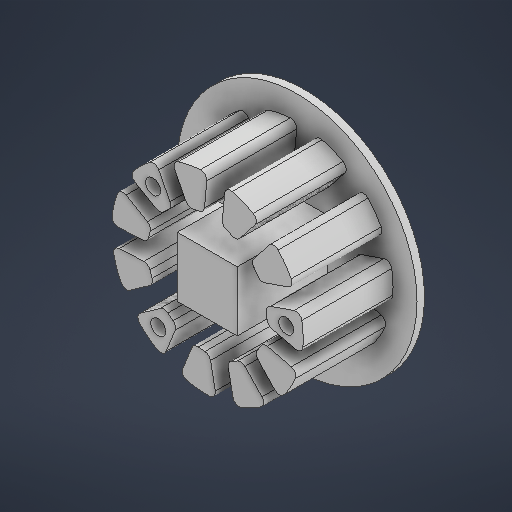
# Autodesk Inventor part: новая сиська 5-26
Saved by Autodesk Inventor 2025 (Build 290162000, 162)
## iProperties
Created: 2025-10-01
Part Number: новая сиська 5-26
Material: Типовые
Document SubType Name: Modeling
Designer: GameHD
Density: 1 g/cm^3
Appearance: По умолчанию
Author: GameHD
Autodesk Inventor part; units mm, degrees
ref_plane "YZ Plane" through (0, 0, 0) normal (1, 0, 0) x (0, 1, 0)
ref_plane "XZ Plane" through (0, 0, 0) normal (0, 1, 0) x (-1, 0, 0)
ref_plane "XY Plane" through (0, 0, 0) normal (0, 0, 1) x (1, 0, 0)
sketch "Эскиз1" plane through (0, 0, 0) normal (0, 0, 1) x (1, 0, 0)
  arc A0 (18.0451, 11.2945) -> (16.7558, 13.0882) centre (1.2512, 0.5834) ccw
  arc A1 (16.735, 15.5731) -> (16.7558, 13.0882) centre (18.3126, 14.3437) ccw
  line L0 (16.735, 15.5731) -> (21.7996, 22.0722)
  arc A2 (24.8522, 22.1935) -> (21.7996, 22.0722) centre (23.3772, 20.8429) ccw
  arc A3 (29.2559, 16.067) -> (24.8522, 22.1935) centre (1.2512, 0.5834) ccw
  arc A4 (28.1681, 13.2122) -> (29.2559, 16.067) centre (27.5056, 15.0993) ccw
  line L1 (28.1681, 13.2122) -> (20.3938, 10.4829)
  arc A5 (18.0451, 11.2945) -> (20.3938, 10.4829) centre (19.7313, 12.37) ccw
  line L2 (-17.9086, -9.4147) -> (-24.6202, -14.1941)
  arc A6 (-27.58, -13.4373) -> (-24.6202, -14.1941) centre (-25.7803, -12.5649) ccw
  arc A7 (-30.0477, -6.3074) -> (-27.58, -13.4373) centre (1.2153, 0.5208) ccw
  arc A8 (-28.189, -3.8829) -> (-30.0477, -6.3074) centre (-28.0938, -5.8806) ccw
  line L3 (-28.189, -3.8829) -> (-19.9588, -3.4908)
  arc A9 (-17.9403, -4.9402) -> (-19.9588, -3.4908) centre (-19.8637, -5.4886) ccw
  arc A10 (-17.9403, -4.9402) -> (-17.2178, -7.0277) centre (1.2153, 0.5208) ccw
  arc A11 (-17.9086, -9.4147) -> (-17.2178, -7.0277) centre (-19.0687, -7.7856) ccw
  line L4 (-9.5011, -18.1766) -> (-12.5634, -25.8259)
  arc A12 (-15.4625, -26.7894) -> (-12.5634, -25.8259) centre (-14.4202, -25.0825) ccw
  arc A13 (-21.3932, -22.1255) -> (-15.4625, -26.7894) centre (1.2153, 0.5208) ccw
  arc A14 (-21.1403, -19.0809) -> (-21.3932, -22.1255) centre (-19.9802, -20.7101) ccw
  line L5 (-21.1403, -19.0809) -> (-14.4286, -14.3016)
  arc A15 (-11.9469, -14.4296) -> (-14.4286, -14.3016) centre (-13.2685, -15.9307) ccw
  arc A16 (-11.9469, -14.4296) -> (-10.2106, -15.7951) centre (1.2153, 0.5208) ccw
  arc A17 (-9.5011, -18.1766) -> (-10.2106, -15.7951) centre (-11.3579, -17.4333) ccw
  line L6 (-15.7668, 13.7891) -> (-22.9023, 17.9088)
  arc A18 (-23.4435, 20.9155) -> (-22.9023, 17.9088) centre (-21.9023, 19.6409) ccw
  arc A19 (-17.983, 26.1221) -> (-23.4435, 20.9155) centre (1.2153, 0.5208) ccw
  arc A20 (-15.0055, 25.4385) -> (-17.983, 26.1221) centre (-16.7831, 24.522) ccw
  line L7 (-15.0055, 25.4385) -> (-11.2299, 18.115)
  arc A21 (-11.7098, 15.6768) -> (-11.2299, 18.115) centre (-13.0076, 17.1985) ccw
  arc A22 (-11.7098, 15.6768) -> (-13.3085, 14.1524) centre (1.2153, 0.5208) ccw
  arc A23 (-15.7668, 13.7891) -> (-13.3085, 14.1524) centre (-14.7668, 15.5211) ccw
  line L8 (21.2475, -7.4256) -> (29.2547, -9.3681)
  arc A24 (30.6211, -12.1006) -> (29.2547, -9.3681) centre (28.7832, -11.3117) ccw
  arc A25 (26.8486, -18.6346) -> (30.6211, -12.1006) centre (1.2153, 0.5208) ccw
  arc A26 (23.7991, -18.8176) -> (26.8486, -18.6346) centre (25.2465, -17.4374) ccw
  line L9 (23.7991, -18.8176) -> (18.1132, -12.8544)
  arc A27 (17.8867, -10.3797) -> (18.1132, -12.8544) centre (19.5607, -11.4742) ccw
  arc A28 (17.8867, -10.3797) -> (18.9912, -8.4668) centre (1.2153, 0.5208) ccw
  arc A29 (21.2475, -7.4256) -> (18.9912, -8.4668) centre (20.776, -9.3692) ccw
  line L10 (22.3636, 4.6661) -> (30.1499, 7.361)
  arc A30 (32.7766, 5.801) -> (30.1499, 7.361) centre (30.8041, 5.471) ccw
  arc A31 (33.1356, -1.7353) -> (32.7766, 5.801) centre (1.2153, 0.5208) ccw
  arc A32 (30.6691, -3.538) -> (33.1356, -1.7353) centre (31.1406, -1.5943) ccw
  line L11 (30.6691, -3.538) -> (22.6619, -1.5954)
  arc A33 (21.1335, 0.3639) -> (22.6619, -1.5954) centre (23.1334, 0.3482) ccw
  arc A34 (21.1335, 0.3639) -> (21.0284, 2.5704) centre (1.2153, 0.5208) ccw
  arc A35 (22.3636, 4.6661) -> (21.0284, 2.5704) centre (23.0178, 2.7761) ccw
  line L12 (-5.8976, 20.864) -> (-9.6731, 28.1875)
  arc A36 (-8.5028, 31.0095) -> (-9.6731, 28.1875) centre (-7.8954, 29.104) ccw
  arc A37 (-1.0943, 32.4374) -> (-8.5028, 31.0095) centre (1.2153, 0.5208) ccw
  arc A38 (1.041, 30.2525) -> (-1.0943, 32.4374) centre (-0.9499, 30.4426) ccw
  line L13 (1.041, 30.2525) -> (0.2578, 22.0503)
  arc A39 (-1.4641, 20.2586) -> (0.2578, 22.0503) centre (-1.7331, 22.2405) ccw
  arc A40 (-1.4641, 20.2586) -> (-3.6331, 19.8406) centre (1.2153, 0.5208) ccw
  arc A41 (-5.8976, 20.864) -> (-3.6331, 19.8406) centre (-4.1199, 21.7804) ccw
  line L14 (2.3087, -21.0022) -> (3.868, -29.0928)
  arc A42 (1.9501, -31.4707) -> (3.868, -29.0928) centre (1.9041, -29.4713) ccw
  arc A43 (-5.5607, -30.7535) -> (1.9501, -31.4707) centre (1.2153, 0.5208) ccw
  arc A44 (-6.9939, -28.0556) -> (-5.5607, -30.7535) centre (-5.1372, -28.7989) ccw
  line L15 (-6.9939, -28.0556) -> (-3.9316, -20.4063)
  arc A45 (-1.7747, -19.1723) -> (-3.9316, -20.4063) centre (-2.0749, -21.1497) ccw
  arc A46 (-1.7747, -19.1723) -> (0.4242, -19.3823) centre (1.2153, 0.5208) ccw
  arc A47 (2.3087, -21.0022) -> (0.4242, -19.3823) centre (0.3448, -21.3807) ccw
  line L16 (-20.2443, 2.5016) -> (-28.4744, 2.1096)
  arc A48 (-30.5552, 4.3464) -> (-28.4744, 2.1096) centre (-28.5696, 4.1073) ccw
  arc A49 (-28.7765, 11.6786) -> (-30.5552, 4.3464) centre (1.2153, 0.5208) ccw
  arc A50 (-25.902, 12.7133) -> (-28.7765, 11.6786) centre (-26.902, 10.9813) ccw
  line L17 (-25.902, 12.7133) -> (-18.7664, 8.5936)
  arc A51 (-17.8519, 6.283) -> (-18.7664, 8.5936) centre (-19.7664, 6.8615) ccw
  arc A52 (-17.8519, 6.283) -> (-18.3727, 4.1363) centre (1.2153, 0.5208) ccw
  arc A53 (-20.2443, 2.5016) -> (-18.3727, 4.1363) centre (-20.3395, 4.4994) ccw
  line L18 (13.7719, -16.9949) -> (19.4572, -22.9575)
  arc A54 (19.1294, -25.9949) -> (19.4572, -22.9575) centre (18.0097, -24.3377) ccw
  arc A55 (12.4232, -29.4522) -> (19.1294, -25.9949) centre (1.2153, 0.5208) ccw
  arc A56 (9.7588, -27.9574) -> (12.4232, -29.4522) centre (11.7227, -27.5789) ccw
  line L19 (9.7588, -27.9574) -> (8.201, -19.8747)
  arc A57 (9.3408, -17.6738) -> (8.201, -19.8747) centre (10.1649, -19.4962) ccw
  arc A58 (9.3408, -17.6738) -> (11.3082, -16.6525) centre (0.9045, 0.9824) ccw
  arc A59 (13.7719, -16.9949) -> (11.3082, -16.6525) centre (12.3244, -18.3751) ccw
  line L20 (6.2299, 21.4801) -> (7.0131, 29.6822)
  arc A60 (9.5233, 31.4235) -> (7.0131, 29.6822) centre (9.0041, 29.4921) ccw
  arc A61 (16.5278, 28.6194) -> (9.5233, 31.4235) centre (1.2153, 0.5208) ccw
  arc A62 (17.1428, 25.6269) -> (16.5278, 28.6194) centre (15.5707, 26.8632) ccw
  line L21 (17.1428, 25.6269) -> (12.0495, 19.1503)
  arc A63 (9.6323, 18.5739) -> (12.0495, 19.1503) centre (10.4774, 20.3866) ccw
  arc A64 (9.6323, 18.5739) -> (7.5816, 19.3949) centre (1.2153, 0.5208) ccw
  arc A65 (6.2299, 21.4801) -> (7.5816, 19.3949) centre (8.2209, 21.29) ccw
  circle A66 centre (1.2153, 0.5208) radius 40
  line L22 (15.3377, 8.6744) -> (15.3377, -7.6327)
  line L23 (15.3377, -7.6327) -> (1.2153, -15.7863)
  line L24 (1.2153, -15.7863) -> (-12.9071, -7.6327)
  line L25 (-12.9071, -7.6327) -> (-12.9071, 8.6744)
  line L26 (-12.9071, 8.6744) -> (1.2153, 16.828)
  line L27 (1.2153, 16.828) -> (15.3377, 8.6744)
  point P0 (0, 0)
  point P1 (1.2153, 0.5208)
  dimension "d9" = 80
  constraints: 132 point on circle, 67 centre point, 56 end point
  measures "d9" diameter of A66
extrude "Выдавливание1" add sketch "Эскиз1" along normal blind 30 contours A0 A1 L0 A2 A3 A4 L1 A5 | L2 A6 A7 A8 L3 A9 A10 A11 | L4 A12 A13 A14 L5 A15 A16 A17 | L6 A18 A19 A20 L7 A21 A22 A23 | L8 A24 A25 A26 L9 A27 A28 A29 | L10 A30 A31 A32 L11 A33 A34 A35 | L12 A36 A37 A38 L13 A39 A40 A41 | L14 A42 A43 A44 L15 A45 A46 A47 | L16 A48 A49 A50 L17 A51 A52 A53 | L18 A54 A55 A56 L19 A57 A58 A59 | L20 A60 A61 A62 L21 A63 A64 A65 | L22 L23 L24 L25 L26 L27
sketch "Эскиз2" plane through (0, 0, 0) normal (0, 0, -1) x (-1, 0, 0)
  line L0 (-15.3377, 8.6744) -> (-1.2153, 16.828) projected
  line L1 (-15.3377, -7.6327) -> (-15.3377, 8.6744) projected
  line L2 (-1.2153, -15.7863) -> (-15.3377, -7.6327) projected
  line L3 (12.9071, -7.6327) -> (-1.2153, -15.7863) projected
  line L4 (12.9071, 8.6744) -> (12.9071, -7.6327) projected
  line L5 (-1.2153, 16.828) -> (12.9071, 8.6744) projected
  arc A0 (-9.5233, 31.4235) -> (-16.5278, 28.6194) centre (-1.2153, 0.5208) ccw projected
  circle A1 centre (-1.2153, 0.5208) radius 40
  point P0 (0, 0)
  dimension "d2" = 80
  constraints: 1 centre point, 1 coincident
  measures "d2" diameter of A1
extrude "Выдавливание2" add sketch "Эскиз2" along normal blind 2.5 contours L0 L5 L4 L3 L2 L1 | A1
sketch "Эскиз3" plane through (0, 0, 30) normal (0, 0, 1) x (1, 0, 0)
  line L0 (15.3377, 8.6744) -> (1.2153, 16.828) projected
  line L1 (1.2153, 16.828) -> (-12.9071, 8.6744) projected
  line L2 (-12.9071, 8.6744) -> (-12.9071, -7.6327) projected
  line L3 (-12.9071, -7.6327) -> (1.2153, -15.7863) projected
  line L4 (1.2153, -15.7863) -> (15.3377, -7.6327) projected
  line L5 (15.3377, -7.6327) -> (15.3377, 8.6744) projected
  arc A0 (-17.983, 26.1221) -> (-23.4435, 20.9155) centre (1.2153, 0.5208) ccw projected
  line L6 (13.7153, -11.9792) -> (-11.2847, -11.9792)
  line L7 (-11.2847, -11.9792) -> (-11.2847, 13.0208)
  line L8 (-11.2847, 13.0208) -> (13.7153, 13.0208)
  line L9 (13.7153, 13.0208) -> (13.7153, -11.9792)
  line L10 (13.7153, -11.9792) -> (-11.2847, 13.0208) construction
  line L11 (-11.2847, -11.9792) -> (13.7153, 13.0208) construction
  point P0 (0, 0)
  dimension "d5" = 25
  dimension "d6" = 25
  constraints: 12 end point, 2 midpoint, 2 parallel, 1 horizontal, 1 perpendicular
  measures "d5" distance of L7.end L8.end
  measures "d6" distance of L6.end L7.end
extrude "Выдавливание3" cut sketch "Эскиз3" against normal up to surface (30 mm away) contours L5 L4 L9 L0 | L8 L1 L0 | L4 L3 L6 | L7 L3 L2 L1
sketch "Эскиз9" plane through (0, 0, 30) normal (0, 0, 1) x (1, 0, 0)
  arc A0 (6.2299, 21.4801) -> (7.5816, 19.3949) centre (8.2209, 21.29) ccw
  arc A1 (6.2299, 21.4801) -> (7.5816, 19.3949) centre (8.2209, 21.29) ccw
  line L0 (12.0495, 19.1503) -> (17.1428, 25.6269)
  line L1 (12.0495, 19.1503) -> (17.1428, 25.6269)
  arc A2 (17.1428, 25.6269) -> (16.5278, 28.6194) centre (15.5707, 26.8632) ccw
  arc A3 (17.1428, 25.6269) -> (16.5278, 28.6194) centre (15.5707, 26.8632) ccw
  arc A4 (16.5278, 28.6194) -> (9.5233, 31.4235) centre (1.2153, 0.5208) ccw
  arc A5 (9.5233, 31.4235) -> (7.0131, 29.6822) centre (9.0041, 29.4921) ccw
  line L2 (7.0131, 29.6822) -> (6.2299, 21.4801)
  arc A6 (-30.5552, 4.3464) -> (-28.4744, 2.1096) centre (-28.5696, 4.1073) ccw
  arc A7 (-30.5552, 4.3464) -> (-28.4744, 2.1096) centre (-28.5696, 4.1073) ccw
  arc A8 (-30.5552, 4.3464) -> (-30.0477, -6.3074) centre (1.2153, 0.5208) ccw
  arc A9 (-27.58, -13.4373) -> (-24.6202, -14.1941) centre (-25.7803, -12.5649) ccw
  arc A10 (-27.58, -13.4373) -> (-24.6202, -14.1941) centre (-25.7803, -12.5649) ccw
  arc A11 (-27.58, -13.4373) -> (-21.3932, -22.1255) centre (1.2153, 0.5208) ccw
  arc A12 (-1.7747, -19.1723) -> (0.4242, -19.3823) centre (1.2153, 0.5208) ccw
  arc A13 (-1.7747, -19.1723) -> (0.4242, -19.3823) centre (1.2153, 0.5208) ccw
  arc A14 (-11.9469, -14.4296) -> (-10.2106, -15.7951) centre (1.2153, 0.5208) ccw
  arc A15 (-11.9469, -14.4296) -> (-10.2106, -15.7951) centre (1.2153, 0.5208) ccw
  arc A16 (-11.9469, -14.4296) -> (-14.4286, -14.3016) centre (-13.2685, -15.9307) ccw
  arc A17 (-11.9469, -14.4296) -> (-14.4286, -14.3016) centre (-13.2685, -15.9307) ccw
  arc A18 (-9.5011, -18.1766) -> (-10.2106, -15.7951) centre (-11.3579, -17.4333) ccw
  arc A19 (-9.5011, -18.1766) -> (-10.2106, -15.7951) centre (-11.3579, -17.4333) ccw
  arc A20 (-1.7747, -19.1723) -> (-3.9316, -20.4063) centre (-2.0749, -21.1497) ccw
  arc A21 (-1.7747, -19.1723) -> (-3.9316, -20.4063) centre (-2.0749, -21.1497) ccw
  arc A22 (2.3087, -21.0022) -> (0.4242, -19.3823) centre (0.3448, -21.3807) ccw
  line L3 (-12.5634, -25.8259) -> (-9.5011, -18.1766)
  line L4 (-12.5634, -25.8259) -> (-9.5011, -18.1766)
  arc A23 (2.3087, -21.0022) -> (0.4242, -19.3823) centre (0.3448, -21.3807) ccw
  arc A24 (-15.4625, -26.7894) -> (-12.5634, -25.8259) centre (-14.4202, -25.0825) ccw
  arc A25 (-15.4625, -26.7894) -> (-12.5634, -25.8259) centre (-14.4202, -25.0825) ccw
  arc A26 (-21.3932, -22.1255) -> (-15.4625, -26.7894) centre (1.2153, 0.5208) ccw
  circle A27 centre (-15.1765, -20.1086) radius 2.48
  line L5 (-14.4286, -14.3016) -> (-21.1403, -19.0809)
  line L6 (-14.4286, -14.3016) -> (-21.1403, -19.0809)
  arc A28 (-21.1403, -19.0809) -> (-21.3932, -22.1255) centre (-19.9802, -20.7101) ccw
  arc A29 (-21.1403, -19.0809) -> (-21.3932, -22.1255) centre (-19.9802, -20.7101) ccw
  arc A30 (9.3408, -17.6738) -> (8.201, -19.8747) centre (10.1649, -19.4962) ccw
  line L7 (8.201, -19.8747) -> (9.7588, -27.9574)
  line L8 (8.201, -19.8747) -> (9.7588, -27.9574)
  arc A31 (9.7588, -27.9574) -> (12.4232, -29.4522) centre (11.7227, -27.5789) ccw
  arc A32 (9.7588, -27.9574) -> (12.4232, -29.4522) centre (11.7227, -27.5789) ccw
  line L9 (3.868, -29.0928) -> (2.3087, -21.0022)
  line L10 (3.868, -29.0928) -> (2.3087, -21.0022)
  arc A33 (1.9501, -31.4707) -> (12.4232, -29.4522) centre (1.2153, 0.5208) ccw
  arc A34 (1.9501, -31.4707) -> (3.868, -29.0928) centre (1.9041, -29.4713) ccw
  arc A35 (1.9501, -31.4707) -> (3.868, -29.0928) centre (1.9041, -29.4713) ccw
  arc A36 (9.3408, -17.6738) -> (8.201, -19.8747) centre (10.1649, -19.4962) ccw
  arc A37 (23.7991, -18.8176) -> (26.8486, -18.6346) centre (25.2465, -17.4374) ccw
  arc A38 (23.7991, -18.8176) -> (26.8486, -18.6346) centre (25.2465, -17.4374) ccw
  line L11 (18.1132, -12.8544) -> (23.7991, -18.8176)
  line L12 (18.1132, -12.8544) -> (23.7991, -18.8176)
  arc A39 (19.1294, -25.9949) -> (26.8486, -18.6346) centre (1.2153, 0.5208) ccw
  arc A40 (26.8486, -18.6346) -> (30.6211, -12.1006) centre (1.2153, 0.5208) ccw
  arc A41 (21.1335, 0.3639) -> (22.6619, -1.5954) centre (23.1334, 0.3482) ccw
  arc A42 (21.1335, 0.3639) -> (22.6619, -1.5954) centre (23.1334, 0.3482) ccw
  arc A43 (22.3636, 4.6661) -> (21.0284, 2.5704) centre (23.0178, 2.7761) ccw
  arc A44 (22.3636, 4.6661) -> (21.0284, 2.5704) centre (23.0178, 2.7761) ccw
  arc A45 (21.1335, 0.3639) -> (21.0284, 2.5704) centre (1.2153, 0.5208) ccw
  arc A46 (21.1335, 0.3639) -> (21.0284, 2.5704) centre (1.2153, 0.5208) ccw
  circle A47 centre (27.5403, 1.6422) radius 2.48
  line L13 (22.6619, -1.5954) -> (30.6691, -3.538)
  arc A48 (30.6691, -3.538) -> (33.1356, -1.7353) centre (31.1406, -1.5943) ccw
  arc A49 (30.6691, -3.538) -> (33.1356, -1.7353) centre (31.1406, -1.5943) ccw
  arc A50 (33.1356, -1.7353) -> (32.7766, 5.801) centre (1.2153, 0.5208) ccw
  line L14 (30.1499, 7.361) -> (22.3636, 4.6661)
  line L15 (30.1499, 7.361) -> (22.3636, 4.6661)
  arc A51 (9.6323, 18.5739) -> (7.5816, 19.3949) centre (1.2153, 0.5208) ccw
  arc A52 (9.6323, 18.5739) -> (7.5816, 19.3949) centre (1.2153, 0.5208) ccw
  arc A53 (9.6323, 18.5739) -> (12.0495, 19.1503) centre (10.4774, 20.3866) ccw
  arc A54 (9.6323, 18.5739) -> (12.0495, 19.1503) centre (10.4774, 20.3866) ccw
  line L16 (7.0131, 29.6822) -> (6.2299, 21.4801)
  arc A55 (9.5233, 31.4235) -> (7.0131, 29.6822) centre (9.0041, 29.4921) ccw
  arc A56 (-1.4641, 20.2586) -> (-3.6331, 19.8406) centre (1.2153, 0.5208) ccw
  arc A57 (-1.4641, 20.2586) -> (-3.6331, 19.8406) centre (1.2153, 0.5208) ccw
  arc A58 (-1.4641, 20.2586) -> (0.2578, 22.0503) centre (-1.7331, 22.2405) ccw
  arc A59 (-1.4641, 20.2586) -> (0.2578, 22.0503) centre (-1.7331, 22.2405) ccw
  line L17 (0.2578, 22.0503) -> (1.041, 30.2525)
  line L18 (0.2578, 22.0503) -> (1.041, 30.2525)
  arc A60 (1.041, 30.2525) -> (-1.0943, 32.4374) centre (-0.9499, 30.4426) ccw
  arc A61 (1.041, 30.2525) -> (-1.0943, 32.4374) centre (-0.9499, 30.4426) ccw
  arc A62 (9.5233, 31.4235) -> (-1.0943, 32.4374) centre (1.2153, 0.5208) ccw
  arc A63 (-11.7098, 15.6768) -> (-13.3085, 14.1524) centre (1.2153, 0.5208) ccw
  arc A64 (-11.7098, 15.6768) -> (-13.3085, 14.1524) centre (1.2153, 0.5208) ccw
  arc A65 (-11.7098, 15.6768) -> (-11.2299, 18.115) centre (-13.0076, 17.1985) ccw
  arc A66 (-11.7098, 15.6768) -> (-11.2299, 18.115) centre (-13.0076, 17.1985) ccw
  line L19 (-8.7847, 10.5208) -> (11.2153, 10.5208)
  line L20 (11.2153, 10.5208) -> (11.2153, -9.4792)
  line L21 (-8.7847, -9.4792) -> (-8.7847, 10.5208)
  line L22 (19.4572, -22.9575) -> (13.7719, -16.9949)
  line L23 (19.4572, -22.9575) -> (13.7719, -16.9949)
  arc A67 (19.1294, -25.9949) -> (19.4572, -22.9575) centre (18.0097, -24.3377) ccw
  arc A68 (19.1294, -25.9949) -> (19.4572, -22.9575) centre (18.0097, -24.3377) ccw
  arc A69 (12.4232, -29.4522) -> (19.1294, -25.9949) centre (1.2153, 0.5208) ccw
  arc A70 (9.3408, -17.6738) -> (11.3082, -16.6525) centre (0.9045, 0.9824) ccw
  arc A71 (9.3408, -17.6738) -> (11.3082, -16.6525) centre (0.9045, 0.9824) ccw
  arc A72 (13.7719, -16.9949) -> (11.3082, -16.6525) centre (12.3244, -18.3751) ccw
  arc A73 (13.7719, -16.9949) -> (11.3082, -16.6525) centre (12.3244, -18.3751) ccw
  arc A74 (-1.0943, 32.4374) -> (-8.5028, 31.0095) centre (1.2153, 0.5208) ccw
  arc A75 (-5.8976, 20.864) -> (-3.6331, 19.8406) centre (-4.1199, 21.7804) ccw
  arc A76 (-8.5028, 31.0095) -> (-9.6731, 28.1875) centre (-7.8954, 29.104) ccw
  arc A77 (-8.5028, 31.0095) -> (-9.6731, 28.1875) centre (-7.8954, 29.104) ccw
  line L24 (-9.6731, 28.1875) -> (-5.8976, 20.864)
  line L25 (-9.6731, 28.1875) -> (-5.8976, 20.864)
  arc A78 (-8.5028, 31.0095) -> (-17.983, 26.1221) centre (1.2153, 0.5208) ccw
  arc A79 (-5.8976, 20.864) -> (-3.6331, 19.8406) centre (-4.1199, 21.7804) ccw
  arc A80 (-15.7668, 13.7891) -> (-13.3085, 14.1524) centre (-14.7668, 15.5211) ccw
  arc A81 (-15.7668, 13.7891) -> (-13.3085, 14.1524) centre (-14.7668, 15.5211) ccw
  line L26 (-11.2299, 18.115) -> (-15.0055, 25.4385)
  line L27 (-11.2299, 18.115) -> (-15.0055, 25.4385)
  circle A82 centre (-16.8714, 19.6817) radius 2.48
  line L28 (-22.9023, 17.9088) -> (-15.7668, 13.7891)
  arc A83 (-15.0055, 25.4385) -> (-17.983, 26.1221) centre (-16.7831, 24.522) ccw
  arc A84 (-15.0055, 25.4385) -> (-17.983, 26.1221) centre (-16.7831, 24.522) ccw
  arc A85 (-17.983, 26.1221) -> (-23.4435, 20.9155) centre (1.2153, 0.5208) ccw
  arc A86 (-23.4435, 20.9155) -> (-22.9023, 17.9088) centre (-21.9023, 19.6409) ccw
  arc A87 (-23.4435, 20.9155) -> (-22.9023, 17.9088) centre (-21.9023, 19.6409) ccw
  arc A88 (-23.4435, 20.9155) -> (-28.7765, 11.6786) centre (1.2153, 0.5208) ccw
  line L29 (-22.9023, 17.9088) -> (-15.7668, 13.7891)
  line L30 (-28.4744, 2.1096) -> (-20.2443, 2.5016)
  line L31 (-28.4744, 2.1096) -> (-20.2443, 2.5016)
  arc A89 (-20.2443, 2.5016) -> (-18.3727, 4.1363) centre (-20.3395, 4.4994) ccw
  arc A90 (-20.2443, 2.5016) -> (-18.3727, 4.1363) centre (-20.3395, 4.4994) ccw
  arc A91 (-28.7765, 11.6786) -> (-30.5552, 4.3464) centre (1.2153, 0.5208) ccw
  arc A92 (-17.8519, 6.283) -> (-18.3727, 4.1363) centre (1.2153, 0.5208) ccw
  arc A93 (-17.8519, 6.283) -> (-18.3727, 4.1363) centre (1.2153, 0.5208) ccw
  arc A94 (-25.902, 12.7133) -> (-28.7765, 11.6786) centre (-26.902, 10.9813) ccw
  arc A95 (-25.902, 12.7133) -> (-28.7765, 11.6786) centre (-26.902, 10.9813) ccw
  arc A96 (-17.8519, 6.283) -> (-18.7664, 8.5936) centre (-19.7664, 6.8615) ccw
  arc A97 (-17.8519, 6.283) -> (-18.7664, 8.5936) centre (-19.7664, 6.8615) ccw
  line L32 (-18.7664, 8.5936) -> (-25.902, 12.7133)
  line L33 (-18.7664, 8.5936) -> (-25.902, 12.7133)
  line L34 (-24.6202, -14.1941) -> (-17.9086, -9.4147)
  line L35 (-24.6202, -14.1941) -> (-17.9086, -9.4147)
  arc A98 (-30.0477, -6.3074) -> (-27.58, -13.4373) centre (1.2153, 0.5208) ccw
  arc A99 (-28.189, -3.8829) -> (-30.0477, -6.3074) centre (-28.0938, -5.8806) ccw
  arc A100 (-28.189, -3.8829) -> (-30.0477, -6.3074) centre (-28.0938, -5.8806) ccw
  line L36 (-19.9588, -3.4908) -> (-28.189, -3.8829)
  line L37 (-19.9588, -3.4908) -> (-28.189, -3.8829)
  arc A101 (-17.9086, -9.4147) -> (-17.2178, -7.0277) centre (-19.0687, -7.7856) ccw
  arc A102 (-17.9086, -9.4147) -> (-17.2178, -7.0277) centre (-19.0687, -7.7856) ccw
  arc A103 (-17.9403, -4.9402) -> (-17.2178, -7.0277) centre (1.2153, 0.5208) ccw
  arc A104 (-17.9403, -4.9402) -> (-17.2178, -7.0277) centre (1.2153, 0.5208) ccw
  arc A105 (-17.9403, -4.9402) -> (-19.9588, -3.4908) centre (-19.8637, -5.4886) ccw
  arc A106 (-17.9403, -4.9402) -> (-19.9588, -3.4908) centre (-19.8637, -5.4886) ccw
  arc A107 (24.4346, 22.5404) -> (16.5278, 28.6194) centre (1.2153, 0.5208) ccw
  arc A108 (16.735, 15.5731) -> (16.7558, 13.0882) centre (18.3126, 14.3437) ccw
  arc A109 (24.4346, 22.5404) -> (21.7996, 22.0722) centre (23.3772, 20.8429) ccw
  arc A110 (18.0451, 11.2945) -> (16.7558, 13.0882) centre (1.2512, 0.5834) ccw
  arc A111 (18.0451, 11.2945) -> (20.3938, 10.4829) centre (19.7313, 12.37) ccw
  arc A112 (28.1681, 13.2122) -> (29.4439, 15.5922) centre (27.5056, 15.0993) ccw
  line L38 (20.3938, 10.4829) -> (28.1681, 13.2122)
  line L39 (21.7996, 22.0722) -> (16.735, 15.5731)
  line L40 (11.2153, -9.4792) -> (-8.7847, -9.4792)
  arc A113 (17.8867, -10.3797) -> (18.1132, -12.8544) centre (19.5607, -11.4742) ccw
  arc A114 (17.8867, -10.3797) -> (18.1132, -12.8544) centre (19.5607, -11.4742) ccw
  arc A115 (-15.4625, -26.7894) -> (-5.5607, -30.7535) centre (1.2153, 0.5208) ccw
  line L41 (-3.9316, -20.4063) -> (-6.9939, -28.0556)
  line L42 (-3.9316, -20.4063) -> (-6.9939, -28.0556)
  arc A116 (-6.9939, -28.0556) -> (-5.5607, -30.7535) centre (-5.1372, -28.7989) ccw
  arc A117 (-6.9939, -28.0556) -> (-5.5607, -30.7535) centre (-5.1372, -28.7989) ccw
  arc A118 (-5.5607, -30.7535) -> (1.9501, -31.4707) centre (1.2153, 0.5208) ccw
  arc A119 (17.8867, -10.3797) -> (18.9912, -8.4668) centre (1.2153, 0.5208) ccw
  arc A120 (17.8867, -10.3797) -> (18.9912, -8.4668) centre (1.2153, 0.5208) ccw
  arc A121 (30.6211, -12.1006) -> (29.2547, -9.3681) centre (28.7832, -11.3117) ccw
  arc A122 (30.6211, -12.1006) -> (29.2547, -9.3681) centre (28.7832, -11.3117) ccw
  arc A123 (21.2475, -7.4256) -> (18.9912, -8.4668) centre (20.776, -9.3692) ccw
  arc A124 (21.2475, -7.4256) -> (18.9912, -8.4668) centre (20.776, -9.3692) ccw
  line L43 (29.2547, -9.3681) -> (21.2475, -7.4256)
  line L44 (29.2547, -9.3681) -> (21.2475, -7.4256)
  line L45 (22.6619, -1.5954) -> (30.6691, -3.538)
  arc A125 (30.6211, -12.1006) -> (33.1356, -1.7353) centre (1.2153, 0.5208) ccw
  arc A126 (32.7766, 5.801) -> (30.1499, 7.361) centre (30.8041, 5.471) ccw
  arc A127 (32.7766, 5.801) -> (24.4346, 22.5404) centre (1.2153, 0.5208) ccw
  arc A128 (32.7766, 5.801) -> (30.1499, 7.361) centre (30.8041, 5.471) ccw
  circle A129 centre (1.2153, 0.5208) radius 40
  circle A130 centre (1.2153, 0.5208) radius 40 projected
  arc A131 (6.2299, 21.4801) -> (7.5816, 19.3949) centre (8.2209, 21.29) ccw projected
  line L46 (7.0131, 29.6822) -> (6.2299, 21.4801) projected
  arc A132 (9.5233, 31.4235) -> (7.0131, 29.6822) centre (9.0041, 29.4921) ccw projected
  arc A133 (16.5278, 28.6194) -> (9.5233, 31.4235) centre (1.2153, 0.5208) ccw projected
  arc A134 (17.1428, 25.6269) -> (16.5278, 28.6194) centre (15.5707, 26.8632) ccw projected
  line L47 (12.0495, 19.1503) -> (17.1428, 25.6269) projected
  arc A135 (9.6323, 18.5739) -> (12.0495, 19.1503) centre (10.4774, 20.3866) ccw projected
  arc A136 (9.6323, 18.5739) -> (7.5816, 19.3949) centre (1.2153, 0.5208) ccw projected
  arc A137 (9.7588, -27.9574) -> (12.4232, -29.4522) centre (11.7227, -27.5789) ccw projected
  line L48 (8.201, -19.8747) -> (9.7588, -27.9574) projected
  arc A138 (9.3408, -17.6738) -> (8.201, -19.8747) centre (10.1649, -19.4962) ccw projected
  arc A139 (9.3408, -17.6738) -> (11.3082, -16.6525) centre (0.9045, 0.9824) ccw projected
  arc A140 (13.7719, -16.9949) -> (11.3082, -16.6525) centre (12.3244, -18.3751) ccw projected
  line L49 (19.4572, -22.9575) -> (13.7719, -16.9949) projected
  arc A141 (19.1294, -25.9949) -> (19.4572, -22.9575) centre (18.0097, -24.3377) ccw projected
  arc A142 (12.4232, -29.4522) -> (19.1294, -25.9949) centre (1.2153, 0.5208) ccw projected
  arc A143 (-25.902, 12.7133) -> (-28.7765, 11.6786) centre (-26.902, 10.9813) ccw projected
  line L50 (-18.7664, 8.5936) -> (-25.902, 12.7133) projected
  arc A144 (-17.8519, 6.283) -> (-18.7664, 8.5936) centre (-19.7664, 6.8615) ccw projected
  arc A145 (-17.8519, 6.283) -> (-18.3727, 4.1363) centre (1.2153, 0.5208) ccw projected
  arc A146 (-20.2443, 2.5016) -> (-18.3727, 4.1363) centre (-20.3395, 4.4994) ccw projected
  line L51 (-28.4744, 2.1096) -> (-20.2443, 2.5016) projected
  arc A147 (-30.5552, 4.3464) -> (-28.4744, 2.1096) centre (-28.5696, 4.1073) ccw projected
  arc A148 (-28.7765, 11.6786) -> (-30.5552, 4.3464) centre (1.2153, 0.5208) ccw projected
  arc A149 (-28.189, -3.8829) -> (-30.0477, -6.3074) centre (-28.0938, -5.8806) ccw projected
  line L52 (-19.9588, -3.4908) -> (-28.189, -3.8829) projected
  arc A150 (-17.9403, -4.9402) -> (-19.9588, -3.4908) centre (-19.8637, -5.4886) ccw projected
  arc A151 (-17.9403, -4.9402) -> (-17.2178, -7.0277) centre (1.2153, 0.5208) ccw projected
  arc A152 (-17.9086, -9.4147) -> (-17.2178, -7.0277) centre (-19.0687, -7.7856) ccw projected
  line L53 (-24.6202, -14.1941) -> (-17.9086, -9.4147) projected
  arc A153 (-27.58, -13.4373) -> (-24.6202, -14.1941) centre (-25.7803, -12.5649) ccw projected
  arc A154 (-30.0477, -6.3074) -> (-27.58, -13.4373) centre (1.2153, 0.5208) ccw projected
  arc A155 (21.2475, -7.4256) -> (18.9912, -8.4668) centre (20.776, -9.3692) ccw projected
  line L54 (29.2547, -9.3681) -> (21.2475, -7.4256) projected
  arc A156 (30.6211, -12.1006) -> (29.2547, -9.3681) centre (28.7832, -11.3117) ccw projected
  arc A157 (26.8486, -18.6346) -> (30.6211, -12.1006) centre (1.2153, 0.5208) ccw projected
  arc A158 (23.7991, -18.8176) -> (26.8486, -18.6346) centre (25.2465, -17.4374) ccw projected
  line L55 (18.1132, -12.8544) -> (23.7991, -18.8176) projected
  arc A159 (17.8867, -10.3797) -> (18.1132, -12.8544) centre (19.5607, -11.4742) ccw projected
  arc A160 (17.8867, -10.3797) -> (18.9912, -8.4668) centre (1.2153, 0.5208) ccw projected
  line L56 (7.8094, -11.9792) -> (13.7153, -8.5694) projected
  line L57 (7.8094, -11.9792) -> (-5.3789, -11.9792) projected
  line L58 (-11.2847, -8.5694) -> (-5.3789, -11.9792) projected
  line L59 (-11.2847, -8.5694) -> (-11.2847, 9.6111) projected
  line L60 (-5.3789, 13.0208) -> (-11.2847, 9.6111) projected
  line L61 (-5.3789, 13.0208) -> (7.8094, 13.0208) projected
  line L62 (13.7153, 9.6111) -> (7.8094, 13.0208) projected
  line L63 (13.7153, 9.6111) -> (13.7153, -8.5694) projected
  arc A161 (28.1681, 13.2122) -> (29.2559, 16.067) centre (27.5056, 15.0993) ccw projected
  line L64 (20.3938, 10.4829) -> (28.1681, 13.2122) projected
  arc A162 (18.0451, 11.2945) -> (20.3938, 10.4829) centre (19.7313, 12.37) ccw projected
  arc A163 (18.0451, 11.2945) -> (16.7558, 13.0882) centre (1.2512, 0.5834) ccw projected
  arc A164 (16.735, 15.5731) -> (16.7558, 13.0882) centre (18.3126, 14.3437) ccw projected
  line L65 (21.7996, 22.0722) -> (16.735, 15.5731) projected
  arc A165 (24.8522, 22.1935) -> (21.7996, 22.0722) centre (23.3772, 20.8429) ccw projected
  arc A166 (29.2559, 16.067) -> (24.8522, 22.1935) centre (1.2512, 0.5834) ccw projected
  arc A167 (-6.9939, -28.0556) -> (-5.5607, -30.7535) centre (-5.1372, -28.7989) ccw projected
  line L66 (-3.9316, -20.4063) -> (-6.9939, -28.0556) projected
  arc A168 (-1.7747, -19.1723) -> (-3.9316, -20.4063) centre (-2.0749, -21.1497) ccw projected
  arc A169 (-1.7747, -19.1723) -> (0.4242, -19.3823) centre (1.2153, 0.5208) ccw projected
  arc A170 (2.3087, -21.0022) -> (0.4242, -19.3823) centre (0.3448, -21.3807) ccw projected
  line L67 (3.868, -29.0928) -> (2.3087, -21.0022) projected
  arc A171 (1.9501, -31.4707) -> (3.868, -29.0928) centre (1.9041, -29.4713) ccw projected
  arc A172 (-5.5607, -30.7535) -> (1.9501, -31.4707) centre (1.2153, 0.5208) ccw projected
  arc A173 (-15.7668, 13.7891) -> (-13.3085, 14.1524) centre (-14.7668, 15.5211) ccw projected
  line L68 (-22.9023, 17.9088) -> (-15.7668, 13.7891) projected
  arc A174 (-23.4435, 20.9155) -> (-22.9023, 17.9088) centre (-21.9023, 19.6409) ccw projected
  arc A175 (-17.983, 26.1221) -> (-23.4435, 20.9155) centre (1.2153, 0.5208) ccw projected
  arc A176 (-15.0055, 25.4385) -> (-17.983, 26.1221) centre (-16.7831, 24.522) ccw projected
  line L69 (-11.2299, 18.115) -> (-15.0055, 25.4385) projected
  arc A177 (-11.7098, 15.6768) -> (-11.2299, 18.115) centre (-13.0076, 17.1985) ccw projected
  arc A178 (-11.7098, 15.6768) -> (-13.3085, 14.1524) centre (1.2153, 0.5208) ccw projected
  arc A179 (-21.1403, -19.0809) -> (-21.3932, -22.1255) centre (-19.9802, -20.7101) ccw projected
  line L70 (-14.4286, -14.3016) -> (-21.1403, -19.0809) projected
  arc A180 (-11.9469, -14.4296) -> (-14.4286, -14.3016) centre (-13.2685, -15.9307) ccw projected
  arc A181 (-11.9469, -14.4296) -> (-10.2106, -15.7951) centre (1.2153, 0.5208) ccw projected
  arc A182 (-9.5011, -18.1766) -> (-10.2106, -15.7951) centre (-11.3579, -17.4333) ccw projected
  line L71 (-12.5634, -25.8259) -> (-9.5011, -18.1766) projected
  arc A183 (-15.4625, -26.7894) -> (-12.5634, -25.8259) centre (-14.4202, -25.0825) ccw projected
  arc A184 (-21.3932, -22.1255) -> (-15.4625, -26.7894) centre (1.2153, 0.5208) ccw projected
  arc A185 (21.1335, 0.3639) -> (22.6619, -1.5954) centre (23.1334, 0.3482) ccw projected
  arc A186 (21.1335, 0.3639) -> (21.0284, 2.5704) centre (1.2153, 0.5208) ccw projected
  arc A187 (22.3636, 4.6661) -> (21.0284, 2.5704) centre (23.0178, 2.7761) ccw projected
  line L72 (30.1499, 7.361) -> (22.3636, 4.6661) projected
  arc A188 (32.7766, 5.801) -> (30.1499, 7.361) centre (30.8041, 5.471) ccw projected
  arc A189 (33.1356, -1.7353) -> (32.7766, 5.801) centre (1.2153, 0.5208) ccw projected
  arc A190 (30.6691, -3.538) -> (33.1356, -1.7353) centre (31.1406, -1.5943) ccw projected
  line L73 (22.6619, -1.5954) -> (30.6691, -3.538) projected
  arc A191 (-1.4641, 20.2586) -> (0.2578, 22.0503) centre (-1.7331, 22.2405) ccw projected
  arc A192 (-1.4641, 20.2586) -> (-3.6331, 19.8406) centre (1.2153, 0.5208) ccw projected
  arc A193 (-5.8976, 20.864) -> (-3.6331, 19.8406) centre (-4.1199, 21.7804) ccw projected
  line L74 (-9.6731, 28.1875) -> (-5.8976, 20.864) projected
  arc A194 (-8.5028, 31.0095) -> (-9.6731, 28.1875) centre (-7.8954, 29.104) ccw projected
  arc A195 (-1.0943, 32.4374) -> (-8.5028, 31.0095) centre (1.2153, 0.5208) ccw projected
  arc A196 (1.041, 30.2525) -> (-1.0943, 32.4374) centre (-0.9499, 30.4426) ccw projected
  line L75 (0.2578, 22.0503) -> (1.041, 30.2525) projected
  circle A197 centre (1.2153, 0.5208) radius 40 projected
  point P0 (0, 0)
  point P1 (1.2221, 0.4307)
  point P2 (0, 0)
  dimension "d26" = 80
  constraints: 253 point on circle, 130 centre point, 92 end point, 1 coincident
  measures "d26" diameter of A129
extrude "Выдавливание6" cut sketch "Эскиз9" against normal up to surface (30 mm away) contours A27 | A47 | A82 | L57 L58 L59 L60 L61 L62 L63 L56
sketch "Эскиз10" plane through (0, 0, 30) normal (0, 0, 1) x (1, 0, 0)
  circle A0 centre (-16.8714, 19.6817) radius 2.48 projected
  circle A1 centre (-15.1765, -20.1086) radius 2.48 projected
  circle A2 centre (27.5403, 1.6422) radius 2.48 projected
  point P0 (0, 0)
extrude "Выдавливание7" cut sketch "Эскиз10" against normal through all
